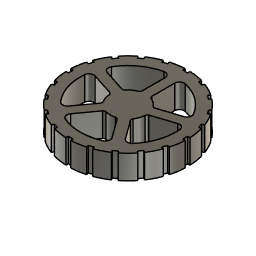
tyre v1 (Autodesk Fusion 360 design; units mm, degrees)
Autodesk Fusion 360 part; units mm, degrees
sketch "Sketch1" plane through (0, 0, 0) normal (0, 0, 1) x (1, 0, 0)
  circle A0 centre (0, 0) radius 25
  line L0 (-2, 7.2284) -> (-2, 19.8997)
  line L1 (2, 19.8997) -> (2, 7.2284)
  line L2 (0, 0) -> (0, 25) construction
  line L3 (-18.3078, 8.0515) -> (-6.2566, 4.1358)
  line L4 (-7.4927, 0.3316) -> (-19.5438, 4.2472)
  line L5 (-13.3148, -14.9237) -> (-5.8668, -4.6723)
  line L6 (-2.6307, -7.0235) -> (-10.0787, -17.2748)
  line L7 (10.0787, -17.2748) -> (2.6307, -7.0235)
  line L8 (5.8668, -4.6723) -> (13.3148, -14.9237)
  line L9 (19.5438, 4.2472) -> (7.4927, 0.3316)
  line L10 (6.2566, 4.1358) -> (18.3078, 8.0515)
  arc A1 (18.3078, 8.0515) -> (2, 19.8997) centre (0, 0) ccw
  arc A2 (6.2566, 4.1358) -> (2, 7.2284) centre (0, 0) ccw
  arc A3 (-2, 7.2284) -> (-6.2566, 4.1358) centre (0, 0) ccw
  arc A4 (-2, 19.8997) -> (-18.3078, 8.0515) centre (0, 0) ccw
  arc A5 (-7.4927, 0.3316) -> (-5.8668, -4.6723) centre (0, 0) ccw
  arc A6 (-2.6307, -7.0235) -> (2.6307, -7.0235) centre (0, 0) ccw
  arc A7 (5.8668, -4.6723) -> (7.4927, 0.3316) centre (0, 0) ccw
  arc A8 (-19.5438, 4.2472) -> (-13.3148, -14.9237) centre (0, 0) ccw
  arc A9 (-10.0787, -17.2748) -> (10.0787, -17.2748) centre (0, 0) ccw
  arc A10 (13.3148, -14.9237) -> (19.5438, 4.2472) centre (0, 0) ccw
  dimension "d4" = 50
  dimension "d5" = 40
  dimension "d7" = 15
  dimension "d9" = 25
  dimension "d10" = 2
  dimension "d12" = 360
  constraint coincident A0.centre L2.start
  constraint concentric A3 A4
  constraint vertical L0
  constraint vertical L1
  constraint coincident A0 L2.end
  constraint vertical L2
  constraint symmetric L0 L1 L2
  constraint concentric A1 A4
  constraint concentric A2 A3
  constraint concentric A3 A5
  constraint concentric A4 A8
  constraint concentric A5 A6
  constraint concentric A6 A7
  constraint concentric A8 A9
  constraint concentric A9 A10
  measures "d4" diameter of A0
  measures "d5" diameter of A4
  measures "d7" diameter of A3
  measures "d9" distance of A0.centre L2.end
  measures "d10" distance of L1 L2
extrude "Extrude1" add sketch "Sketch1" along normal blind 10
sketch "Sketch2" plane through (0, 0, 0) normal (0, 0, 1) x (1, 0, 0)
  line L0 (2.0567, 1.9) -> (-2.0567, 1.9)
  line L1 (-2.0567, -1.9) -> (2.0567, -1.9)
  line L2 (2.0567, 1.9) -> (-2.0567, -1.9) construction
  line L3 (-2.0567, 1.9) -> (2.0567, -1.9) construction
  arc A0 (-2.0567, 1.9) -> (-2.0567, -1.9) centre (0, 0) ccw
  arc A1 (2.0567, -1.9) -> (2.0567, 1.9) centre (0, 0) ccw
  line L4 (0, 0) -> (0, 1.9) construction
  dimension "d17" = 3.8
  dimension "d18" = 2.8
  constraint horizontal L0
  constraint parallel L0 L1
  constraint coincident L2 A0.centre
  constraint coincident L3 A0.centre
  constraint coincident A0.centre A1.centre
  constraint concentric A0 A1
  constraint midpoint L0 L4.end
  measures "d17" distance of L0.end L1.start
  measures "d18" radius of A1
extrude "Extrude2" cut sketch "Sketch2" along normal blind 10
ref_plane "WorkPlane1" through (0, 30, 0) normal (0, 1, 0) x (0, 0, 1)
sketch "Sketch3" plane through (0, 30, 0) normal (0, 1, 0) x (1, 0, 0)
  line L0 (-1, 0) -> (1, 0)
  line L1 (1, 0) -> (1, -10)
  line L2 (1, -10) -> (-1, -10)
  line L3 (-1, -10) -> (-1, 0)
  line L4 (0, 0) -> (0, -10) construction
  line L5 (0, 0) -> (7.4642, 0) construction
  dimension "d23" = 2
  dimension "d24" = 10
  constraint horizontal L0
  constraint vertical L1
  constraint horizontal L2
  constraint vertical L3
  constraint coincident L4.start L5.start
  constraint perpendicular L0 L4
  constraint symmetric L1 L3 L4
  constraint perpendicular L4 L5
  constraint collinear L0 L5
  measures "d23" distance of L0.start L0.end
  measures "d24" distance of L0.start L2.end
emboss "Emboss1" depth -1 profiles "Sketch3" section 1 onto face at (24.9689, -1.2461, 6.6667)
fillet "Fillet1" radius 2 10 edges at (2, 19.8997, 5) (18.3078, 8.0515, 5) (-18.3078, 8.0515, 5) (-19.5438, 4.2472, 5) (-2, 19.8997, 5) (19.5438, 4.2472, 5) (13.3148, -14.9237, 5) (-13.3148, -14.9237, 5) (-10.0787, -17.2748, 5) (10.0787, -17.2748, 5)
fillet "Fillet2" radius 1 10 edges at (-6.2566, 4.1358, 5) (-2, 7.2284, 5) (2, 7.2284, 5) (6.2566, 4.1358, 5) (7.4927, 0.3316, 5) (5.8668, -4.6723, 5) (2.6307, -7.0235, 5) (-2.6307, -7.0235, 5) (-5.8668, -4.6723, 5) (-7.4927, 0.3316, 5)
pattern_circular "C-Pattern1" count 20 over 360 about axis through (0, 0, 1.75) along (0, 0, 1) of "Emboss1"
sketch "Sketch5" plane through (0, 0, 10) normal (0, 0, 1) x (-1, 0, 0)
  line L0 (-2.0567, 1.9) -> (2.0567, 1.9)
  arc A0 (2.0567, -1.9) -> (2.0567, 1.9) centre (0, 0) ccw
  line L1 (2.0567, -1.9) -> (-2.0567, -1.9)
  arc A1 (-2.0567, 1.9) -> (-2.0567, -1.9) centre (0, 0) ccw
  line L2 (17.309, -3.5211) -> (8.1818, -0.5555)
  arc A2 (7.4919, 0.349) -> (8.1818, -0.5555) centre (8.4908, 0.3956) ccw
  arc A3 (7.4919, 0.349) -> (6.2662, 4.1212) centre (0, 0) ccw
  arc A4 (6.2927, 5.2585) -> (6.2662, 4.1212) centre (7.1017, 4.6707) ccw
  line L3 (6.2927, 5.2585) -> (11.9336, 13.0226)
  arc A5 (15.0574, 13.1634) -> (11.9336, 13.0226) centre (13.5517, 11.847) ccw
  arc A6 (19.9189, -1.7989) -> (15.0574, 13.1634) centre (0, 0) ccw
  arc A7 (17.309, -3.5211) -> (19.9189, -1.7989) centre (17.927, -1.619) ccw
  arc A8 (-17.1721, -10.2527) -> (-4.4444, -19.4999) centre (0, 0) ccw
  arc A9 (-16.0729, -7.3253) -> (-17.1721, -10.2527) centre (-15.4549, -9.2275) ccw
  line L4 (-16.0729, -7.3253) -> (-6.9457, -4.3597)
  arc A10 (-5.8559, -4.686) -> (-6.9457, -4.3597) centre (-6.6367, -5.3108) ccw
  arc A11 (-5.8559, -4.686) -> (-2.6471, -7.0173) centre (0, 0) ccw
  arc A12 (-2, -7.953) -> (-2.6471, -7.0173) centre (-3, -7.953) ccw
  line L5 (-2, -7.953) -> (-2, -17.5499)
  arc A13 (-4.4444, -19.4999) -> (-2, -17.5499) centre (-4, -17.5499) ccw
  line L6 (2, -17.5499) -> (2, -7.953)
  arc A14 (2.6471, -7.0173) -> (2, -7.953) centre (3, -7.953) ccw
  arc A15 (2.6471, -7.0173) -> (5.8559, -4.686) centre (0, 0) ccw
  arc A16 (6.9457, -4.3597) -> (5.8559, -4.686) centre (6.6367, -5.3108) ccw
  line L7 (6.9457, -4.3597) -> (16.0729, -7.3253)
  arc A17 (17.1721, -10.2527) -> (16.0729, -7.3253) centre (15.4549, -9.2275) ccw
  arc A18 (4.4444, -19.4999) -> (17.1721, -10.2527) centre (0, 0) ccw
  arc A19 (2, -17.5499) -> (4.4444, -19.4999) centre (4, -17.5499) ccw
  line L8 (8.6976, 15.3738) -> (3.0566, 7.6097)
  arc A20 (1.9832, 7.2331) -> (3.0566, 7.6097) centre (2.2476, 8.1975) ccw
  arc A21 (1.9832, 7.2331) -> (-1.9832, 7.2331) centre (0, 0) ccw
  arc A22 (-3.0566, 7.6097) -> (-1.9832, 7.2331) centre (-2.2476, 8.1975) ccw
  line L9 (-3.0566, 7.6097) -> (-8.6976, 15.3738)
  arc A23 (-7.8661, 18.3881) -> (-8.6976, 15.3738) centre (-7.0795, 16.5493) ccw
  arc A24 (7.8661, 18.3881) -> (-7.8661, 18.3881) centre (0, 0) ccw
  arc A25 (8.6976, 15.3738) -> (7.8661, 18.3881) centre (7.0795, 16.5493) ccw
  line L10 (-11.9336, 13.0226) -> (-6.2927, 5.2585)
  arc A26 (-6.2662, 4.1212) -> (-6.2927, 5.2585) centre (-7.1017, 4.6707) ccw
  arc A27 (-6.2662, 4.1212) -> (-7.4919, 0.349) centre (0, 0) ccw
  arc A28 (-8.1818, -0.5555) -> (-7.4919, 0.349) centre (-8.4908, 0.3956) ccw
  line L11 (-8.1818, -0.5555) -> (-17.309, -3.5211)
  arc A29 (-19.9189, -1.7989) -> (-17.309, -3.5211) centre (-17.927, -1.619) ccw
  arc A30 (-15.0574, 13.1634) -> (-19.9189, -1.7989) centre (0, 0) ccw
  arc A31 (-11.9336, 13.0226) -> (-15.0574, 13.1634) centre (-13.5517, 11.847) ccw
  line L12 (8.67, 23.4485) -> (8.3232, 22.5105)
  arc A32 (8.3232, 22.5105) -> (6.4977, 23.1037) centre (0, 0) ccw
  line L13 (6.4977, 23.1037) -> (6.7684, 24.0663)
  arc A33 (-6.7684, -24.0663) -> (-0.9997, -24.98) centre (0, 0) ccw
  line L14 (-0.9997, -24.98) -> (-0.9597, -23.9808)
  arc A34 (-0.9597, -23.9808) -> (0.9597, -23.9808) centre (0, 0) ccw
  line L15 (0.9597, -23.9808) -> (0.9997, -24.98)
  arc A35 (0.9997, -24.98) -> (6.7684, -24.0663) centre (0, 0) ccw
  line L16 (6.7684, -24.0663) -> (6.4977, -23.1037)
  arc A36 (6.4977, -23.1037) -> (8.3232, -22.5105) centre (0, 0) ccw
  line L17 (8.3232, -22.5105) -> (8.67, -23.4485)
  arc A37 (8.67, -23.4485) -> (13.8741, -20.7969) centre (0, 0) ccw
  line L18 (13.8741, -20.7969) -> (13.3191, -19.965)
  arc A38 (13.3191, -19.965) -> (14.872, -18.8368) centre (0, 0) ccw
  line L19 (14.872, -18.8368) -> (15.4917, -19.6216)
  arc A39 (15.4917, -19.6216) -> (19.6216, -15.4917) centre (0, 0) ccw
  line L20 (19.6216, -15.4917) -> (18.8368, -14.872)
  arc A40 (18.8368, -14.872) -> (19.965, -13.3191) centre (0, 0) ccw
  line L21 (19.965, -13.3191) -> (20.7969, -13.8741)
  arc A41 (20.7969, -13.8741) -> (23.4485, -8.67) centre (0, 0) ccw
  line L22 (23.4485, -8.67) -> (22.5105, -8.3232)
  arc A42 (22.5105, -8.3232) -> (23.1037, -6.4977) centre (0, 0) ccw
  line L23 (23.1037, -6.4977) -> (24.0663, -6.7684)
  arc A43 (24.0663, -6.7684) -> (24.98, -0.9997) centre (0, 0) ccw
  line L24 (24.98, -0.9997) -> (23.9808, -0.9597)
  arc A44 (23.9808, -0.9597) -> (23.9808, 0.9597) centre (0, 0) ccw
  line L25 (23.9808, 0.9597) -> (24.98, 0.9997)
  arc A45 (24.98, 0.9997) -> (24.0663, 6.7684) centre (0, 0) ccw
  line L26 (24.0663, 6.7684) -> (23.1037, 6.4977)
  arc A46 (23.1037, 6.4977) -> (22.5105, 8.3232) centre (0, 0) ccw
  line L27 (22.5105, 8.3232) -> (23.4485, 8.67)
  arc A47 (23.4485, 8.67) -> (20.7969, 13.8741) centre (0, 0) ccw
  line L28 (20.7969, 13.8741) -> (19.965, 13.3191)
  arc A48 (19.965, 13.3191) -> (18.8368, 14.872) centre (0, 0) ccw
  line L29 (18.8368, 14.872) -> (19.6216, 15.4917)
  arc A49 (19.6216, 15.4917) -> (15.4917, 19.6216) centre (0, 0) ccw
  line L30 (15.4917, 19.6216) -> (14.872, 18.8368)
  arc A50 (14.872, 18.8368) -> (13.3191, 19.965) centre (0, 0) ccw
  line L31 (13.3191, 19.965) -> (13.8741, 20.7969)
  arc A51 (13.8741, 20.7969) -> (8.67, 23.4485) centre (0, 0) ccw
  circle A52 centre (0, 0) radius 7.5
  line L32 (-8.67, -23.4485) -> (-8.3232, -22.5105)
  arc A53 (-8.3232, -22.5105) -> (-6.4977, -23.1037) centre (0, 0) ccw
  line L33 (-6.4977, -23.1037) -> (-6.7684, -24.0663)
  arc A54 (6.7684, 24.0663) -> (0.9997, 24.98) centre (0, 0) ccw
  line L34 (0.9997, 24.98) -> (0.9597, 23.9808)
  arc A55 (0.9597, 23.9808) -> (-0.9597, 23.9808) centre (0, 0) ccw
  line L35 (-0.9597, 23.9808) -> (-0.9997, 24.98)
  arc A56 (-0.9997, 24.98) -> (-6.7684, 24.0663) centre (0, 0) ccw
  line L36 (-6.7684, 24.0663) -> (-6.4977, 23.1037)
  arc A57 (-6.4977, 23.1037) -> (-8.3232, 22.5105) centre (0, 0) ccw
  line L37 (-8.3232, 22.5105) -> (-8.67, 23.4485)
  arc A58 (-8.67, 23.4485) -> (-13.8741, 20.7969) centre (0, 0) ccw
  line L38 (-13.8741, 20.7969) -> (-13.3191, 19.965)
  arc A59 (-13.3191, 19.965) -> (-14.872, 18.8368) centre (0, 0) ccw
  line L39 (-14.872, 18.8368) -> (-15.4917, 19.6216)
  arc A60 (-15.4917, 19.6216) -> (-19.6216, 15.4917) centre (0, 0) ccw
  line L40 (-19.6216, 15.4917) -> (-18.8368, 14.872)
  arc A61 (-18.8368, 14.872) -> (-19.965, 13.3191) centre (0, 0) ccw
  line L41 (-19.965, 13.3191) -> (-20.7969, 13.8741)
  arc A62 (-20.7969, 13.8741) -> (-23.4485, 8.67) centre (0, 0) ccw
  line L42 (-23.4485, 8.67) -> (-22.5105, 8.3232)
  arc A63 (-22.5105, 8.3232) -> (-23.1037, 6.4977) centre (0, 0) ccw
  line L43 (-23.1037, 6.4977) -> (-24.0663, 6.7684)
  arc A64 (-24.0663, 6.7684) -> (-24.98, 0.9997) centre (0, 0) ccw
  line L44 (-24.98, 0.9997) -> (-23.9808, 0.9597)
  arc A65 (-23.9808, 0.9597) -> (-23.9808, -0.9597) centre (0, 0) ccw
  line L45 (-23.9808, -0.9597) -> (-24.98, -0.9997)
  arc A66 (-24.98, -0.9997) -> (-24.0663, -6.7684) centre (0, 0) ccw
  line L46 (-24.0663, -6.7684) -> (-23.1037, -6.4977)
  arc A67 (-23.1037, -6.4977) -> (-22.5105, -8.3232) centre (0, 0) ccw
  line L47 (-22.5105, -8.3232) -> (-23.4485, -8.67)
  arc A68 (-23.4485, -8.67) -> (-20.7969, -13.8741) centre (0, 0) ccw
  line L48 (-20.7969, -13.8741) -> (-19.965, -13.3191)
  arc A69 (-19.965, -13.3191) -> (-18.8368, -14.872) centre (0, 0) ccw
  line L49 (-18.8368, -14.872) -> (-19.6216, -15.4917)
  arc A70 (-19.6216, -15.4917) -> (-15.4917, -19.6216) centre (0, 0) ccw
  line L50 (-15.4917, -19.6216) -> (-14.872, -18.8368)
  arc A71 (-14.872, -18.8368) -> (-13.3191, -19.965) centre (0, 0) ccw
  line L51 (-13.3191, -19.965) -> (-13.8741, -20.7969)
  arc A72 (-13.8741, -20.7969) -> (-8.67, -23.4485) centre (0, 0) ccw
  dimension "d36" = 15
  constraint concentric A0 A52
  measures "d36" diameter of A52
extrude "Extrude3" add sketch "Sketch5" against normal blind 1 contours L0 A0 L1 A1 | A3 A11 A15 A21 A27 A52
sketch "Sketch6" plane through (0, 0, 0) normal (0, 0, -1) x (1, 0, 0)
  line L0 (8.3232, -22.5105) -> (8.67, -23.4485)
  arc A0 (8.67, -23.4485) -> (13.8741, -20.7969) centre (0, 0) ccw
  line L1 (13.8741, -20.7969) -> (13.3191, -19.965)
  arc A1 (13.3191, -19.965) -> (14.872, -18.8368) centre (0, 0) ccw
  line L2 (14.872, -18.8368) -> (15.4917, -19.6216)
  arc A2 (15.4917, -19.6216) -> (19.6216, -15.4917) centre (0, 0) ccw
  line L3 (19.6216, -15.4917) -> (18.8368, -14.872)
  arc A3 (18.8368, -14.872) -> (19.965, -13.3191) centre (0, 0) ccw
  line L4 (19.965, -13.3191) -> (20.7969, -13.8741)
  arc A4 (20.7969, -13.8741) -> (23.4485, -8.67) centre (0, 0) ccw
  line L5 (23.4485, -8.67) -> (22.5105, -8.3232)
  arc A5 (22.5105, -8.3232) -> (23.1037, -6.4977) centre (0, 0) ccw
  line L6 (23.1037, -6.4977) -> (24.0663, -6.7684)
  arc A6 (24.0663, -6.7684) -> (24.98, -0.9997) centre (0, 0) ccw
  line L7 (24.98, -0.9997) -> (23.9808, -0.9597)
  arc A7 (23.9808, -0.9597) -> (23.9808, 0.9597) centre (0, 0) ccw
  line L8 (23.9808, 0.9597) -> (24.98, 0.9997)
  arc A8 (24.98, 0.9997) -> (24.0663, 6.7684) centre (0, 0) ccw
  line L9 (24.0663, 6.7684) -> (23.1037, 6.4977)
  arc A9 (23.1037, 6.4977) -> (22.5105, 8.3232) centre (0, 0) ccw
  line L10 (22.5105, 8.3232) -> (23.4485, 8.67)
  arc A10 (23.4485, 8.67) -> (20.7969, 13.8741) centre (0, 0) ccw
  line L11 (20.7969, 13.8741) -> (19.965, 13.3191)
  arc A11 (19.965, 13.3191) -> (18.8368, 14.872) centre (0, 0) ccw
  line L12 (18.8368, 14.872) -> (19.6216, 15.4917)
  arc A12 (19.6216, 15.4917) -> (15.4917, 19.6216) centre (0, 0) ccw
  line L13 (15.4917, 19.6216) -> (14.872, 18.8368)
  arc A13 (14.872, 18.8368) -> (13.3191, 19.965) centre (0, 0) ccw
  line L14 (13.3191, 19.965) -> (13.8741, 20.7969)
  arc A14 (13.8741, 20.7969) -> (8.67, 23.4485) centre (0, 0) ccw
  line L15 (8.67, 23.4485) -> (8.3232, 22.5105)
  arc A15 (8.3232, 22.5105) -> (6.4977, 23.1037) centre (0, 0) ccw
  line L16 (6.4977, 23.1037) -> (6.7684, 24.0663)
  arc A16 (6.7684, 24.0663) -> (0.9997, 24.98) centre (0, 0) ccw
  line L17 (0.9997, 24.98) -> (0.9597, 23.9808)
  arc A17 (0.9597, 23.9808) -> (-0.9597, 23.9808) centre (0, 0) ccw
  line L18 (-0.9597, 23.9808) -> (-0.9997, 24.98)
  arc A18 (-0.9997, 24.98) -> (-6.7684, 24.0663) centre (0, 0) ccw
  line L19 (-6.7684, 24.0663) -> (-6.4977, 23.1037)
  arc A19 (-6.4977, 23.1037) -> (-8.3232, 22.5105) centre (0, 0) ccw
  line L20 (-8.3232, 22.5105) -> (-8.67, 23.4485)
  arc A20 (-8.67, 23.4485) -> (-13.8741, 20.7969) centre (0, 0) ccw
  line L21 (-13.8741, 20.7969) -> (-13.3191, 19.965)
  arc A21 (-13.3191, 19.965) -> (-14.872, 18.8368) centre (0, 0) ccw
  line L22 (-14.872, 18.8368) -> (-15.4917, 19.6216)
  arc A22 (-15.4917, 19.6216) -> (-19.6216, 15.4917) centre (0, 0) ccw
  line L23 (-19.6216, 15.4917) -> (-18.8368, 14.872)
  arc A23 (-18.8368, 14.872) -> (-19.965, 13.3191) centre (0, 0) ccw
  line L24 (-19.965, 13.3191) -> (-20.7969, 13.8741)
  arc A24 (-20.7969, 13.8741) -> (-23.4485, 8.67) centre (0, 0) ccw
  line L25 (-23.4485, 8.67) -> (-22.5105, 8.3232)
  arc A25 (-22.5105, 8.3232) -> (-23.1037, 6.4977) centre (0, 0) ccw
  line L26 (-23.1037, 6.4977) -> (-24.0663, 6.7684)
  arc A26 (-24.0663, 6.7684) -> (-24.98, 0.9997) centre (0, 0) ccw
  line L27 (-24.98, 0.9997) -> (-23.9808, 0.9597)
  arc A27 (-23.9808, 0.9597) -> (-23.9808, -0.9597) centre (0, 0) ccw
  line L28 (-23.9808, -0.9597) -> (-24.98, -0.9997)
  arc A28 (-24.98, -0.9997) -> (-24.0663, -6.7684) centre (0, 0) ccw
  line L29 (-24.0663, -6.7684) -> (-23.1037, -6.4977)
  arc A29 (-23.1037, -6.4977) -> (-22.5105, -8.3232) centre (0, 0) ccw
  line L30 (-22.5105, -8.3232) -> (-23.4485, -8.67)
  arc A30 (-23.4485, -8.67) -> (-20.7969, -13.8741) centre (0, 0) ccw
  line L31 (-20.7969, -13.8741) -> (-19.965, -13.3191)
  arc A31 (-19.965, -13.3191) -> (-18.8368, -14.872) centre (0, 0) ccw
  line L32 (-18.8368, -14.872) -> (-19.6216, -15.4917)
  arc A32 (-19.6216, -15.4917) -> (-15.4917, -19.6216) centre (0, 0) ccw
  line L33 (-15.4917, -19.6216) -> (-14.872, -18.8368)
  arc A33 (-14.872, -18.8368) -> (-13.3191, -19.965) centre (0, 0) ccw
  line L34 (-13.3191, -19.965) -> (-13.8741, -20.7969)
  arc A34 (-13.8741, -20.7969) -> (-8.67, -23.4485) centre (0, 0) ccw
  line L35 (-8.67, -23.4485) -> (-8.3232, -22.5105)
  arc A35 (-8.3232, -22.5105) -> (-6.4977, -23.1037) centre (0, 0) ccw
  line L36 (-6.4977, -23.1037) -> (-6.7684, -24.0663)
  arc A36 (-6.7684, -24.0663) -> (-0.9997, -24.98) centre (0, 0) ccw
  line L37 (-0.9997, -24.98) -> (-0.9597, -23.9808)
  arc A37 (-0.9597, -23.9808) -> (0.9597, -23.9808) centre (0, 0) ccw
  line L38 (0.9597, -23.9808) -> (0.9997, -24.98)
  arc A38 (0.9997, -24.98) -> (6.7684, -24.0663) centre (0, 0) ccw
  line L39 (6.7684, -24.0663) -> (6.4977, -23.1037)
  arc A39 (6.4977, -23.1037) -> (8.3232, -22.5105) centre (0, 0) ccw
  line L40 (-2.0567, 1.9) -> (2.0567, 1.9)
  arc A40 (2.0567, -1.9) -> (2.0567, 1.9) centre (0, 0) ccw
  line L41 (2.0567, -1.9) -> (-2.0567, -1.9)
  arc A41 (-2.0567, 1.9) -> (-2.0567, -1.9) centre (0, 0) ccw
  arc A42 (-19.9189, -1.7989) -> (-17.309, -3.5211) centre (-17.927, -1.619) ccw
  arc A43 (-15.0574, 13.1634) -> (-19.9189, -1.7989) centre (0, 0) ccw
  arc A44 (-11.9336, 13.0226) -> (-15.0574, 13.1634) centre (-13.5517, 11.847) ccw
  line L42 (-11.9336, 13.0226) -> (-6.2927, 5.2585)
  arc A45 (-6.2662, 4.1212) -> (-6.2927, 5.2585) centre (-7.1017, 4.6707) ccw
  arc A46 (-6.2662, 4.1212) -> (-7.4919, 0.349) centre (0, 0) ccw
  arc A47 (-8.1818, -0.5555) -> (-7.4919, 0.349) centre (-8.4908, 0.3956) ccw
  line L43 (-8.1818, -0.5555) -> (-17.309, -3.5211)
  arc A48 (2, -17.5499) -> (4.4444, -19.4999) centre (4, -17.5499) ccw
  line L44 (2, -17.5499) -> (2, -7.953)
  arc A49 (2.6471, -7.0173) -> (2, -7.953) centre (3, -7.953) ccw
  arc A50 (2.6471, -7.0173) -> (5.8559, -4.686) centre (0, 0) ccw
  arc A51 (6.9457, -4.3597) -> (5.8559, -4.686) centre (6.6367, -5.3108) ccw
  line L45 (6.9457, -4.3597) -> (16.0729, -7.3253)
  arc A52 (17.1721, -10.2527) -> (16.0729, -7.3253) centre (15.4549, -9.2275) ccw
  arc A53 (4.4444, -19.4999) -> (17.1721, -10.2527) centre (0, 0) ccw
  arc A54 (-4.4444, -19.4999) -> (-2, -17.5499) centre (-4, -17.5499) ccw
  arc A55 (-17.1721, -10.2527) -> (-4.4444, -19.4999) centre (0, 0) ccw
  arc A56 (-16.0729, -7.3253) -> (-17.1721, -10.2527) centre (-15.4549, -9.2275) ccw
  line L46 (-16.0729, -7.3253) -> (-6.9457, -4.3597)
  arc A57 (-5.8559, -4.686) -> (-6.9457, -4.3597) centre (-6.6367, -5.3108) ccw
  arc A58 (-5.8559, -4.686) -> (-2.6471, -7.0173) centre (0, 0) ccw
  arc A59 (-2, -7.953) -> (-2.6471, -7.0173) centre (-3, -7.953) ccw
  line L47 (-2, -7.953) -> (-2, -17.5499)
  arc A60 (-7.8661, 18.3881) -> (-8.6976, 15.3738) centre (-7.0795, 16.5493) ccw
  arc A61 (7.8661, 18.3881) -> (-7.8661, 18.3881) centre (0, 0) ccw
  arc A62 (8.6976, 15.3738) -> (7.8661, 18.3881) centre (7.0795, 16.5493) ccw
  line L48 (8.6976, 15.3738) -> (3.0566, 7.6097)
  arc A63 (1.9832, 7.2331) -> (3.0566, 7.6097) centre (2.2476, 8.1975) ccw
  arc A64 (1.9832, 7.2331) -> (-1.9832, 7.2331) centre (0, 0) ccw
  arc A65 (-3.0566, 7.6097) -> (-1.9832, 7.2331) centre (-2.2476, 8.1975) ccw
  line L49 (-3.0566, 7.6097) -> (-8.6976, 15.3738)
  arc A66 (15.0574, 13.1634) -> (11.9336, 13.0226) centre (13.5517, 11.847) ccw
  arc A67 (19.9189, -1.7989) -> (15.0574, 13.1634) centre (0, 0) ccw
  arc A68 (17.309, -3.5211) -> (19.9189, -1.7989) centre (17.927, -1.619) ccw
  line L50 (17.309, -3.5211) -> (8.1818, -0.5555)
  arc A69 (7.4919, 0.349) -> (8.1818, -0.5555) centre (8.4908, 0.3956) ccw
  arc A70 (7.4919, 0.349) -> (6.2662, 4.1212) centre (0, 0) ccw
  arc A71 (6.2927, 5.2585) -> (6.2662, 4.1212) centre (7.1017, 4.6707) ccw
  line L51 (6.2927, 5.2585) -> (11.9336, 13.0226)
  circle A72 centre (0, 0) radius 5
  dimension "d40" = 10
  constraint coincident A0.centre A1.centre
  measures "d40" diameter of A72
extrude "Extrude4" add sketch "Sketch6" along normal blind 7 contours A72
equation "dia = 50 mm"
equation "cthik = 10 mm"
equation "thik = 10 mm"
equation "d4 = dia"
equation "d5 = dia - cthik"
equation "incircle = 15 mm"
equation "d7 = incircle"
equation "recThik = 4 mm"
equation "d9 = dia / 2"
equation "d10 = recThik / 2"
equation "d13 = thik"
equation "mrlength = 5.6 mm"
equation "mrwidth = 3.8 mm"
equation "d17 = mrwidth"
equation "d18 = mrlength / 2"
equation "d19 = thik"
equation "d21 = dia / 2 + 5 mm"
equation "patwidth = 2 mm"
equation "d23 = patwidth"
equation "d24 = thik"
equation "d25 = patDepth"
equation "patDepth = -1 mm"
equation "d36 = incircle"
equation "sideDepth = 1 mm"
equation "d38 = -sideDepth"
equation "d40 = extendedCircleRadius"
equation "extendedCircleRadius = 10 mm"
